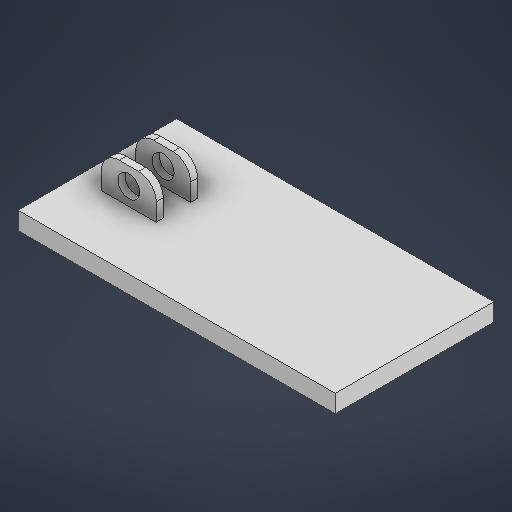
# Autodesk Inventor part: base
Saved by Autodesk Inventor 2027 (Build 310192060, 192F)
## iProperties
Created: 2026-10-07
Part Number: base
Material: Genérico
Document SubType Name: Modeling
Designer: guisg
Density: 1 g/cm^3
Appearance: Padrão
Author: guisg
Autodesk Inventor part; units mm, degrees
ref_plane "YZ Plane" through (0, 0, 0) normal (1, 0, 0) x (0, 1, 0)
ref_plane "XZ Plane" through (0, 0, 0) normal (0, 1, 0) x (-1, 0, 0)
ref_plane "XY Plane" through (0, 0, 0) normal (0, 0, 1) x (1, 0, 0)
sketch "Esboço1" plane through (0, 0, 0) normal (0, 1, 0) x (-1, 0, 0)
  line L0 (0, 0) -> (-180, 0)
  line L1 (-180, 0) -> (-180, -90)
  line L2 (-180, -90) -> (0, -90)
  line L3 (0, -90) -> (0, 0)
  dimension "d25" = 180
  constraints: 8 end point, 2 horizontal, 2 perpendicular
  measures "d25" distance of L1.end L2.end
extrude "Extrusão1" add sketch "Esboço1" along normal blind 20
chamfer "Chanfro1" distance 10 angle 45 4 edges at (90, 0, 0) (180, 0, -45) (90, 0, -90) (0, 0, -45)
fillet "Arredondamento1" radius 5 4 edges at (90, 0, -80) (10, 0, -45) (90, 0, -10) (170, 0, -45)
sketch "Esboço4" plane through (0, 20, 0) normal (0, 1, 0) x (1, 0, 0)
  line L0 (0, 90) -> (0, 0) projected
  line L1 (171.4645, 8.5355) -> (8.5355, 8.5355) projected
  line L2 (30, 52.75) -> (45.1, 52.75)
  line L3 (45.1, 52.75) -> (45.1, 56.75)
  line L4 (45.1, 56.75) -> (14.1, 56.75)
  line L5 (14.1, 56.75) -> (14.1, 52.75)
  line L6 (14.1, 52.75) -> (30, 52.75)
  line L7 (12.0711, 77.9289) -> (12.0711, 12.0711) projected
  line L8 (30, 37.25) -> (45.1, 37.25)
  line L9 (45.1, 37.25) -> (45.1, 33.25)
  line L10 (45.1, 33.25) -> (14.1, 33.25)
  line L11 (14.1, 33.25) -> (14.1, 37.25)
  line L12 (14.1, 37.25) -> (30, 37.25)
  dimension "d49" = 15.1
  dimension "d50" = 4
  dimension "d51" = 31
  dimension "d52" = 4
  constraints: 20 end point, 8 perpendicular, 2 horizontal, 1 point on line
  measures "d49" distance of L2.start L2.end
  measures "d50" distance of L2.end L3.end
  measures "d51" distance of L3.end L4.end
  measures "d52" distance of L8.end L9.end
extrude "Extrusão4" add sketch "Esboço4" along normal blind 20
fillet "Arredondamento4" radius 10 4 edges at (45.1, 40, -35.25) (45.1, 40, -54.75) (14.1, 40, -54.75) (14.1, 40, -35.25)
sketch "Esboço6" plane through (14.1, 20, -33.25) normal (0, 0, 1) x (1, 0, 0)
  line L0 (21, 20) -> (10, 20) projected
  line L1 (31, 0) -> (0, 0) projected
  line L2 (0, 0) -> (0, 10) projected
  circle A0 centre (15.5, 10) radius 6.15
  point P0 (-14.1, -20)
  dimension "d54" = 12.3
  constraints: 1 centre point
  measures "d54" diameter of A0
extrude "Extrusão6" cut sketch "Esboço6" against normal blind 24
